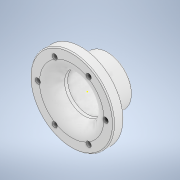
# Autodesk Inventor part: 5201_Bias_Coil_Mounting_Flange_MPSv2_v2
Saved by Autodesk Inventor 2021 (Build 250183000, 183)
## iProperties
Created: 2020-11-11
Part Number: 5201_Bias_Coil_Mounting_Flange_MPSv2_v2
Material: Acetal Resin, White
Document SubType Name: Modeling
Designer: Admin
Density: 1.425 g/cm^3
Appearance: Smooth - White
Author: Admin
Autodesk Inventor part; units mm, degrees
ref_plane "YZ Plane" through (0, 0, 0) normal (1, 0, 0) x (0, 1, 0)
ref_plane "XZ Plane" through (0, 0, 0) normal (0, 1, 0) x (-1, 0, 0)
ref_plane "XY Plane" through (0, 0, 0) normal (0, 0, 1) x (1, 0, 0)
sketch "Sketch1" plane through (0, 0, 0) normal (0, 0, 1) x (1, 0, 0)
  point P0 (0, 0)
sketch "Sketch2" plane through (0, 0, 0) normal (0, 0, 1) x (1, 0, 0)
  circle A0 centre (0, 0) radius 18.8587
  circle A1 centre (0, 0) radius 20.6375
  dimension "d0" = 37.7174
  dimension "d1" = 41.275
  constraints: 2 centre point, 2 coincident
  measures "d0" diameter of A0
  measures "d1" diameter of A1
extrude "Extrusion1" add sketch "Sketch2" along normal blind 5
sketch "Sketch3" plane through (0, 0, 0) normal (0, 0, -1) x (-1, 0, 0)
  circle A0 centre (0, 0) radius 20.6375
  circle A1 centre (0, 0) radius 23.1375
  dimension "d4" = 46.275
  constraints: 2 centre point, 2 coincident
  measures "d4" diameter of A1
extrude "Extrusion2" add sketch "Sketch3" along normal blind 20 and the other way blind 5
sketch "Sketch5" plane through (0, 0, 5) normal (0, 0, 1) x (1, 0, 0)
  circle A0 centre (0, 0) radius 18.8587
  circle A1 centre (0, 0) radius 40
  dimension "d14" = 80
  constraints: 2 centre point, 2 coincident
  measures "d14" diameter of A1
extrude "Extrusion4" add sketch "Sketch5" along normal blind 10
sketch "Sketch6" plane through (0, 0, 5) normal (0, 0, -1) x (-1, 0, 0)
  line L0 (0, 0) -> (-40, 0)
  circle A0 centre (0, 0) radius 40 projected
  line L1 (0, 0) -> (-30, 0)
  circle A1 centre (0, 0) radius 30
  line L2 (0, 0) -> (30, 0)
  line L3 (0, 0) -> (15, -25.9808)
  line L4 (0, 0) -> (-15, -25.9808)
  line L5 (0, 0) -> (-15, 25.9808)
  line L6 (0, 0) -> (15, 25.9808)
  circle A2 centre (-30, 0) radius 2.5
  circle A3 centre (-15, 25.9808) radius 2.5
  circle A4 centre (15, 25.9808) radius 2.5
  circle A5 centre (30, 0) radius 2.5
  circle A6 centre (15, -25.9808) radius 2.5
  circle A7 centre (-15, -25.9808) radius 2.5
  circle A8 centre (-32.5, 0) radius 2.5
  circle A9 centre (-16.25, -28.1458) radius 2.5
  circle A10 centre (16.25, -28.1458) radius 2.5
  circle A11 centre (32.5, 0) radius 2.5
  circle A12 centre (16.25, 28.1458) radius 2.5
  circle A13 centre (-16.25, 28.1458) radius 2.5
  dimension "d18" = 5
  dimension "d19" = 5
  dimension "d20" = 5
  dimension "d21" = 5
  dimension "d22" = 5
  dimension "d23" = 5
  dimension "d17" = 30
  dimension "d26" = 5
  dimension "d27" = 5
  dimension "d28" = 5
  dimension "d29" = 5
  dimension "d30" = 5
  dimension "d31" = 5
  constraints: 14 end point, 6 centre point, 6 coincident, 4 point on line, 3 horizontal alignment, 2 horizontal, 26 other
  measures "d17" distance of L1.start L1.end
  measures "d26" diameter of A8
  measures "d27" diameter of A9
  measures "d28" diameter of A10
  measures "d29" diameter of A11
  measures "d30" diameter of A12
  measures "d31" diameter of A13
extrude "Extrusion6" cut sketch "Sketch6" against normal blind 10 contours A8 A2 L0 | L0 A2 A8 | A11 A5 | A10 A6 | A9 A7 | A13 A3 | A12 A4 | A2 A8 L0 | L0 A8 A2 | A11 A5 | A10 A6 | A9 A7 | A3 A13 | A4 A12
fillet "Fillet2" radius 5 1 edges at (23.1375, 0, 5)
fillet "Fillet3" radius 12 1 edges at (-18.8587, 0, 15)
fillet "Fillet4" radius 1 2 edges at (-40, 0, 5) (-40, 0, 15)
fillet "Fillet5" radius 1 2 edges at (20.6375, 0, -20) (23.1375, 0, -20)
body "Solid1"
